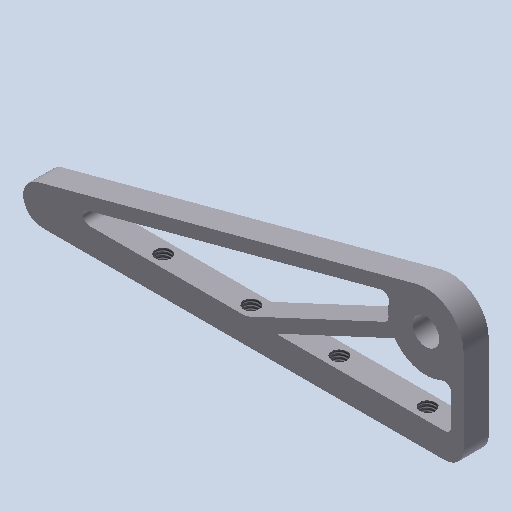
# Autodesk Inventor part: PLATE,TURNBUCKLE,TENSIONER,CHAIN
Saved by Autodesk Inventor 2025.2 (Build 292293000, 293)
## iProperties
Category: _
Manager: _
ILogicPurgeVersion: 0.0.0.0
OnSaveVersion: 3.4.3.0
OnSaveAssembly: COREAutomationManager
Created: 2025-01-30
Part Number: PLATE,TURNBUCKLE,TENSIONER,CHAIN
Checked By: 00
Engr Approved By: _
User Status: Work In Process
Material: Aluminum, 7075-T6
Description: STANDARD (mm)
Document SubType Name: Modeling
Mfg Approved By: John.Thibert
Designer: John.Thibert
Manufacturer: Standard
Standards Organization: Custom
Density: 2.81 g/cm^3
Appearance: Metal-AL-6061 (Flat)
Mass: 25.5619 g
Surface Area: 63.6817 cm^2
Volume: 9.09677 cm^3
CN_MASS: 0.03
CN_SERVICEABLE: _
FIRST_DESCRIPTION: _
SECOND_DESCRIPTION: _
THIRD_DESCRIPTION: _
ModelCat: Uncategorized
MaterialName: Aluminum, 7075-T6
Subject: _
Author: John.Thibert
Keywords: -
Revision Number: A
Autodesk Inventor part; units mm, degrees
ref_plane "YZ Plane" through (0, 0, 0) normal (1, 0, 0) x (0, 1, 0)
ref_plane "XZ Plane" through (0, 0, 0) normal (0, 1, 0) x (-1, 0, 0)
ref_plane "XY Plane" through (0, 0, 0) normal (0, 0, 1) x (1, 0, 0)
sketch "Sketch2" plane through (0, 0, 0) normal (0, 0, 1) x (1, 0, 0)
  line L0 (43.5797, 34.8995) -> (-52.0289, 9.3637)
  line L1 (-50.8, 0) -> (50.8, 0)
  line L2 (55.5625, 4.7625) -> (55.5625, 25.6971)
  arc A0 (55.5625, 25.6971) -> (43.5797, 34.8995) centre (46.0375, 25.6971) ccw
  arc A1 (-52.0289, 9.3637) -> (-50.8, 0) centre (-50.8, 4.7625) ccw
  arc A2 (50.8, 0) -> (55.5625, 4.7625) centre (50.8, 4.7625) ccw
  arc A3 (43.5797, 34.8995) -> (37.5399, 30.0001) centre (46.0375, 25.6971) ccw construction
  line L3 (-51.0083, 6.35) -> (37.5399, 30.0001)
  line L4 (52.3875, 18.5976) -> (52.3875, 6.35)
  arc A4 (52.3875, 18.5976) -> (55.5625, 25.6971) centre (46.0375, 25.6971) ccw construction
  arc A5 (37.5399, 30.0001) -> (52.3875, 18.5976) centre (46.0375, 25.6971) ccw
  line L5 (0.6896, 6.35) -> (36.8433, 23.2087)
  line L6 (52.3875, 6.35) -> (-51.0083, 6.35)
  line L7 (38.1719, 20.3251) -> (8.2023, 6.35)
  point P0 (0, 0)
  point P1 (55.5625, 38.1)
  point P2 (-87.0876, 0)
  point P3 (55.5625, 0)
  point P4 (0, 0)
  point P5 (31.5247, 6.35)
  point P6 (34.848, 29.2811)
  dimension "d0" = 38.1
  dimension "d2" = 9.525
  dimension "d3" = 4.7625
  dimension "d7" = 3.175
  dimension "d28" = 101.6
  dimension "d29" = 3.175
  dimension "d31" = 3.175
  dimension "d32" = 25
  dimension "d33" = 6.35
  constraints: 16 end point, 15 point on circle, 8 point on line, 6 centre point, 6 tangent, 2 horizontal, 2 midpoint, 2 parallel, 1 coincident, 1 equal radius, 1 perpendicular
  measures "d0" distance from line of L1 point (55.562, 38.1)
  measures "d2" radius of A0
  measures "d3" radius of A1
  measures "d7" distance between parallel lines of L0 L3
  measures "d28" distance of L1.start L1.end
  measures "d29" distance between parallel lines of L2 L4
  measures "d31" distance between parallel lines of L5 L7
  measures "d32" angle of L6 L7
  measures "d33" distance between parallel lines of L1 L6
extrude "Extrusion1" add sketch "Sketch2" along normal mid plane 6.35 contours A0 L2 A2 L1 A1 L0 | L5 A5 L7 L6
fillet "Fillet1" radius 1.5875 5 edges at (37.5399, 30.0001, 0) (36.8433, 23.2087, 0) (52.3875, 18.5976, 0) (52.3875, 6.35, 0) (-51.0083, 6.35, 0)
sketch "Sketch4" plane through (0, 0, 3.175) normal (0, 0, 1) x (1, 0, 0)
  arc A0 (55.5625, 25.6971) -> (43.5797, 34.8995) centre (46.0375, 25.6971) ccw construction
  point P0 (0, 0)
  constraints: 1 coincident
hole "Hole2" at (46.0375, 25.6971, 3.175) direction (0, 0, -1) diameter 6.7564 end through all clearance for "Flat Head Machine Screw (82)" size "1/4" standard "Ansi Unified Screw Threads"
sketch "Sketch5" plane through (-50.8, 0, 3.175) normal (0, -1, 0) x (1, 0, 0)
  line L0 (106.3625, -6.35) -> (106.3625, 0) construction
  line L1 (0, 0) -> (101.6, 0) construction
  point P0 (50.8, -3.175)
  point P1 (94.0898, -3.1755)
  dimension "d35" = 12.2727
  dimension "d36" = 3.1755
  measures "d35" distance from line of L0 point (94.09, -3.175)
  measures "d36" distance from line of point (94.09, -3.175) L1
hole "Hole3" at (43.2898, 0, -0.0005) direction (0, 1, 0) diameter 3.9624 depth 6.35 tip angle 118 thread size "10-32 UNF" class "2B" standard "ANSI Unified Screw Threads"
pattern_linear "Rectangular Pattern2" count 5 spacing 22.225 along (-1, 0, 0) of "Hole3"
equation "\"d29\" = d7"
body "Solid1"
